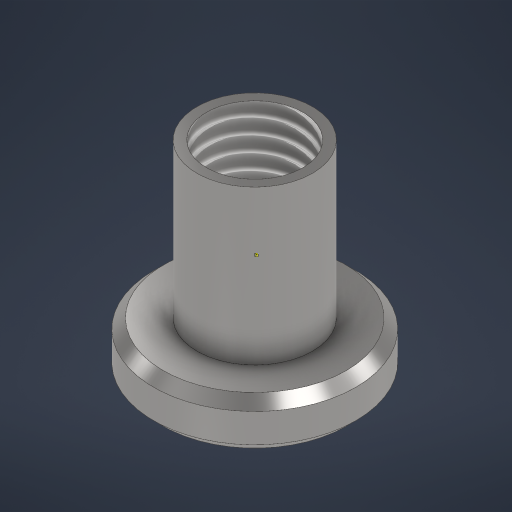
# Autodesk Inventor part: M5-D6-8mm
Saved by Autodesk Inventor 2024.3 (Build 283343000, 343)
## iProperties
Created: 2025-01-10
Part Number: M5-D6-8mm
Material: 스테인리스스틸
Document SubType Name: Modeling
Designer: ASUS
Density: 8 g/cm^3
Appearance: 반연마
Author: ASUS
Autodesk Inventor part; units mm, degrees
ref_plane "YZ Plane" through (0, 0, 0) normal (1, 0, 0) x (0, 1, 0)
ref_plane "XZ Plane" through (0, 0, 0) normal (0, 1, 0) x (-1, 0, 0)
ref_plane "XY Plane" through (0, 0, 0) normal (0, 0, 1) x (1, 0, 0)
sketch "스케치1" plane through (0, 0, 0) normal (0, 0, 1) x (1, 0, 0)
  line L0 (0, 0) -> (0, 2.5)
  line L1 (0, 2.5) -> (5.25, 2.5)
  line L2 (5.25, 2.5) -> (5.25, 0)
  line L3 (5.25, 0) -> (0, 0)
  line L4 (0, 2.5) -> (0, 10.5)
  line L5 (0, 10.5) -> (3, 10.5)
  line L6 (3, 10.5) -> (3, 2.5)
  line L7 (3, 2.5) -> (0, 2.5)
  dimension "d0" = 2.5
  dimension "d1" = 5.25
  dimension "d2" = 8
  dimension "d3" = 3
  constraints: 16 end point, 4 parallel, 2 perpendicular, 2 vertical
  measures "d0" distance of L0.start L0.end
  measures "d1" distance of L0.end L1.end
  measures "d2" distance of L0.end L4.end
  measures "d3" distance of L4.end L5.end
revolve "회전1" add sketch "스케치1" angle 360 about axis through (0, 2.5, 0) along (0, 1, 0)
sketch "스케치2" plane through (0, 10.5, 0) normal (0, 1, 0) x (1, 0, 0)
  circle A0 centre (0, 0) radius 3 projected
  circle A1 centre (0, 0) radius 2.5
  dimension "d5" = 5
  constraints: 1 centre point, 1 coincident
  measures "d5" diameter of A1
extrude "돌출1" cut sketch "스케치2" against normal up to surface (8 mm away) contours A1
thread "스레드1" size "M5x0.8" class "6H" standard "ANSI Metric M Profile" full length
chamfer "모따기1" distance 0.5 angle 45 2 edges at (-5.25, 0, 0) (-5.25, 2.5, 0)
sketch "스케치3" plane through (0, 0, 0) normal (0, -1, 0) x (1, 0, 0)
  circle A0 centre (0, 0) radius 2.5 projected
  line L0 (1.7321, 0) -> (0.866, -1.5)
  line L1 (0.866, -1.5) -> (-0.866, -1.5)
  line L2 (-0.866, -1.5) -> (-1.7321, 0)
  line L3 (-1.7321, 0) -> (-0.866, 1.5)
  line L4 (-0.866, 1.5) -> (0.866, 1.5)
  line L5 (0.866, 1.5) -> (1.7321, 0)
  dimension "d13" = 3
  constraints: 12 end point, 1 coincident, 13 other
  measures "d13" distance between parallel lines of L1 L4
extrude "돌출2" cut sketch "스케치3" against normal blind 2 contours L0 L1 L2 L3 L4 L5
chamfer "모따기2" distance 0.5 angle 45 6 edges at (1.299, 0, 0.75) (1.299, 0, -0.75) (0, 0, -1.5) (-1.299, 0, -0.75) (-1.299, 0, 0.75) (0, 0, 1.5)
